Autodesk Fusion 360 part; units mm, degrees
note: some values were not read from the file. Set by a fixed rule: the direction of a hole.
(part 2 of 2)
hole "Bohrung1" at (0, 4, 0) direction (0, 0, 1) diameter 2.175 end through all
thread "Gewinde1" "ISO Metric profile 2.6 M2.6x0.45 6H" major diameter 2.675 minor diameter 2.1754 pitch 0.45 angle 60 resizes the face on face at (0.1083, 5.0821, 3.1667)
extrude "Extrusion3" cut sketch "Skizze1" along normal blind 3.5 contours L0 L4 L5 L6 | L1 L11 L12 L13
extrude "Extrusion7" add sketch "Skizze1" along normal up to surface (4.7 mm away) from surface at 4.8 contours L2 L7 L8 L9
chamfer "Fase1" distance 1.5 angle 45 1 edges at (0, -1.5, 4.8)
sketch "Skizze4" plane through (0, 0, 9.5) normal (0, 0, 1) x (-1, 0, 0)
  line L0 (-18.366, 1.5) -> (-7.95, -16.5411)
  line L1 (7.95, -16.5411) -> (18.366, 1.5)
  line L2 (7.95, -16.5411) -> (18.366, 1.5)
  line L3 (7.95, -16.5411) -> (18.366, 1.5)
  line L4 (14.9474, 1.5787) -> (13.2679, -1.3301)
  line L5 (13.2679, -1.3301) -> (15.866, -2.8301)
  line L6 (18.366, 1.5) -> (-18.366, 1.5)
  line L7 (1.8167, -13) -> (7.95, -16.5411)
  line L8 (-7.95, -16.5411) -> (-1.8167, -13)
  line L9 (-1.8167, -13) -> (1.8167, -13)
  circle A0 centre (0, -4) radius 1.0877
  line L10 (0, 0) -> (0, -13)
  line L11 (-13.2679, -1.3301) -> (-15.866, -2.8301)
  line L12 (-14.9474, 1.5787) -> (-13.2679, -1.3301)
  line L13 (18.366, 1.5) -> (-18.366, 1.5)
  dimension "d62" = 3
  dimension "d63" = 5
  constraint parallel L2 L4
  constraint coincident L2 L5.end
  constraint perpendicular L2 L5
  constraint coincident L10.start origin
  constraint midpoint L9 L10.end
  constraint symmetric L4.start L10 L12.start
  constraint symmetric L4.end L10 L11.start
  constraint symmetric L5.end L10 L11.end
  measures "d62" distance of L4.end L5.end
  measures "d63" distance of L1.end L5
extrude "Extrusion8" cut sketch "Skizze4" against normal through all contours L0 L6 L11 L12 L13 | L1 L2 L3 L4 L5 L6 L13
fillet "Abrundung6" radius 2 2 edges at (-13.2679, 1.3301, 4.75) (13.2679, 1.3301, 4.75)
sketch "Skizze5" plane through (0, 0, 0) normal (0, 0, -1) x (1, 0, 0)
  line L0 (-15, -2.3301) -> (-15.866, -2.8301)
  line L1 (-15.866, -2.8301) -> (-14.7, -4.8497)
  line L2 (-14.7, -4.8497) -> (-7.512, -0.6997)
  line L3 (-7.512, -0.6997) -> (-0.762, -12.3911)
  line L4 (-0.762, -12.3911) -> (-1.8167, -13)
  line L5 (-1.8167, -13) -> (1.8167, -13)
  line L6 (1.8167, -13) -> (0.762, -12.3911)
  line L7 (0.762, -12.3911) -> (7.512, -0.6997)
  line L8 (7.512, -0.6997) -> (14.7, -4.8497)
  line L9 (14.7, -4.8497) -> (15.866, -2.8301)
  line L10 (15.866, -2.8301) -> (15, -2.3301)
  arc A0 (14.0915, 0) -> (15, -2.3301) centre (16, -0.5981) ccw
  line L11 (14.0915, 0) -> (-14.0915, 0)
  arc A1 (-15, -2.3301) -> (-14.0915, 0) centre (-16, -0.5981) ccw
  circle A2 centre (0, -4) radius 1.0877
  arc A3 (-5.5, 0) -> (-2.5, 0) centre (-4, 0) ccw
  line L12 (0, 0) -> (0, -2.9123)
  arc A4 (2.5, 0) -> (5.5, 0) centre (4, 0) ccw
  dimension "d81" = 3
  dimension "d82" = 8
  constraint coincident L11 A3.centre
  constraint coincident L11 A3.end
  constraint coincident L11 A3.start
  constraint coincident L12.start origin
  constraint coincident A2 L12.end
  constraint perpendicular L11 L12
  constraint symmetric A3.end L12 A4.start
  constraint symmetric A3.start L12 A4.end
  constraint symmetric A3 L12 A4
  measures "d81" diameter of A3
  measures "d82" distance of A3.centre A4.centre
extrude "Extrusion9" cut sketch "Skizze5" against normal blind 4.8 contours L11 A3 | L11 A4
ref_plane "Arbeitsebene2" through (0, 2, 0) normal (0, 1, 0) x (0, 0, 1)
sketch "Skizze6" plane through (0, 2, 0) normal (0, 1, 0) x (1, 0, 0)
  line L0 (-14.5736, -9.5) -> (14.5736, -9.5)
  line L1 (-10.1, -7.2) -> (-7.6, -7.2)
  line L2 (-7.6, -7.2) -> (-5.3, -9.5)
  arc A0 (-10.1, -7.45) -> (-10.3, -8.5123) centre (-10.1, -8) ccw
  line L3 (-10.1, -7.45) -> (-10.1, -7.2)
  line L4 (-10.3, -8.5123) -> (-10.3, -9.5)
  dimension "d86" = 1.1
  dimension "d89" = 2.5
  dimension "d90" = 45
  dimension "d102" = 10.1
  dimension "d103" = 1.5
  dimension "d104" = 0.2
  dimension "d105" = 2.3
  constraint coincident L0 L2.end
  constraint vertical L3
  constraint coincident L0 L4.end
  constraint perpendicular L0 L4
  constraint horizontal L1
  constraint coincident A0.centre L3
  measures "d86" diameter of A0
  measures "d89" distance of L1.start L1.end
  measures "d90" angle of L1 L2
  measures "d102" distance of origin L3
  measures "d103" distance of L0 A0.centre
  measures "d104" distance of L3 L4
  measures "d105" distance of L0 L1
extrude "Extrusion10" cut sketch "Skizze6" along normal blind 6.2 and the other way blind 0.2
fillet "Abrundung7" radius 0.2 2 edges at (-10.1, 5, 7.45) (-10.3, 5, 8.5123)
chamfer "Fase3" distance 0.4 angle 60 1 edges at (-10.3, 5, 9.5) measured on face at (5.7939, 6.4585, 9.5)
mirror "Spiegeln3" about plane through (0, 0, 0) normal (1, 0, 0) of "Extrusion10", "Abrundung7", "Fase3"
equation "d7 = 0deg 0'"
equation "d13 = 118deg 0'"
equation "d31 = ( 5 * 2.54 ) * 1 mm + 0.8 mm"
equation "d35 = 0deg 0'"
equation "d58 = 6.5 mm - 1.7 mm"
equation "d60 = 0deg 0'"
equation "d64 = 0deg 0'"
equation "d84 = 0deg 0'"
equation "d93 = 0deg 0'"
equation "d99 = 0deg 0'"
equation "d107 = 60deg 0'"
